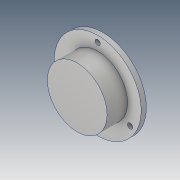
# Autodesk Inventor part: Motor mesh
Saved by Autodesk Inventor 2019 (Build 230136000, 136)
## iProperties
Created: 2019-09-03
Part Number: Motor mesh
Material: Alumínio 6061
Document SubType Name: Modeling
Designer: Daniel Regner
Mass: 47.5475 g
Surface Area: 59.2819 cm^2
Volume: 17.6102 cm^3
Density: 2.7 g/cm^3
Appearance: Alumínio - Plano
Author: Daniel Regner
Autodesk Inventor part; units mm, degrees
ref_plane "YZ Plane" through (0, 0, 0) normal (1, 0, 0) x (0, 1, 0)
ref_plane "XZ Plane" through (0, 0, 0) normal (0, 1, 0) x (-1, 0, 0)
ref_plane "XY Plane" through (0, 0, 0) normal (0, 0, 1) x (1, 0, 0)
sketch "Esboço1" plane through (0, 0, 0) normal (0, 0, 1) x (1, 0, 0)
  circle A0 centre (0, 0) radius 25.5
  dimension "d0" = 51
  constraints: 1 centre point, 1 coincident
  measures "d0" diameter of A0
extrude "Extrusão1" add sketch "Esboço1" along normal blind 3
sketch "Esboço2" plane through (0, 0, 3) normal (0, 0, 1) x (1, 0, 0)
  circle A0 centre (0, 0) radius 17.5
  circle A1 centre (-0.0486, 21.9399) radius 1.5
  line L0 (-0.0486, 17.4999) -> (-0.0486, -17.4999)
  dimension "d3" = 35
  dimension "d4" = 21.94
  dimension "d5" = 3
  constraints: 2 centre point, 2 end point, 2 point on circle, 1 coincident, 1 point on line, 1 vertical
  measures "d3" diameter of A0
  measures "d4" distance of point (0, 0) A1.centre
  measures "d5" diameter of A1
extrude "Extrusão2" add sketch "Esboço2" along normal blind 12 contours A0 L0 | L0 A0
sketch "Esboço3" plane through (0, 0, 3) normal (0, 0, 1) x (1, 0, 0)
  circle A0 centre (0, 0) radius 17.5 projected
  point P0 (0, 21.94)
  point P1 (-19.0006, -10.97)
  point P2 (19.0006, -10.97)
  dimension "d8" = 21.94
  dimension "d11" = 360
  constraints: 4 other
  measures "d8" distance of A0.centre point (0, 21.94)
hole "Furo1" at (0, 21.94, 3) at (-19.0006, -10.97, 3) at (19.0006, -10.97, 3) direction (0, 0, -1) diameter 3 end through all
